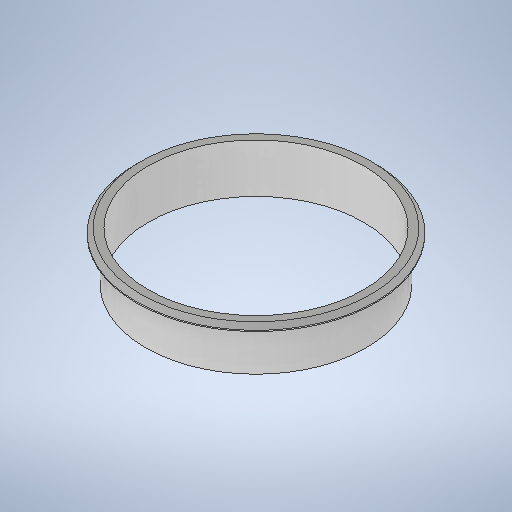
# Autodesk Inventor part: Bevel V1
Saved by Autodesk Inventor 2025.1 (Build 291241020, 241B)
## iProperties
Created: 2024-08-09
Part Number: Bevel V1
Material: Generic
Document SubType Name: Modeling
Designer: balmo
Density: 1 g/cm^3
Appearance: Default
Author: balmo
## iProperties of the stored document Bevel V1_3DPrint.ipt
Created: 2024-08-09
Part Number: Bevel V1_3DPrint
Material: Generic
Document SubType Name: Modeling
Designer: balmo
Density: 1 g/cm^3
Appearance: Default
Author: balmo
Autodesk Inventor part; units mm, degrees
ref_plane "YZ Plane" through (0, 0, 0) normal (1, 0, 0) x (0, 1, 0)
ref_plane "XZ Plane" through (0, 0, 0) normal (0, 1, 0) x (-1, 0, 0)
ref_plane "XY Plane" through (0, 0, 0) normal (0, 0, 1) x (1, 0, 0)
sketch "Sketch1" plane through (0, 0, 0) normal (0, 1, 0) x (-1, 0, 0)
  circle A0 centre (0, 0) radius 62.865
  circle A1 centre (0, 0) radius 69.85
  circle A2 centre (0, 0) radius 64.4525
  dimension "d0" = 125.73
  dimension "d1" = 139.7
  dimension "d2" = 1.5875
  constraints: 3 centre point, 3 coincident
  measures "d0" diameter of A0
  measures "d1" diameter of A1
  measures "d2" radial gap between concentric circles of A2 A0
extrude "Extrusion1" add sketch "Sketch1" along normal blind 28.575 contours A2
extrude "Extrusion2" add sketch "Sketch1" along normal blind 3.175 contours A1
chamfer "Chamfer1" distance 2.54 angle 45 1 edges at (69.85, 0, 0)
body "Solid1"
